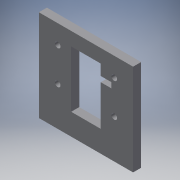
# Autodesk Inventor part: Camera holder plate
Saved by Autodesk Inventor 2018 (Build 220112000, 112)
## iProperties
Created: 2018-06-25
Part Number: Camera holder plate
Material: Generic
Document SubType Name: Modeling
Designer: Ajith Thomas
Density: 1 g/cm^3
Appearance: Default
Author: Ajith Thomas
Autodesk Inventor part; units mm, degrees
ref_plane "YZ Plane" through (0, 0, 0) normal (1, 0, 0) x (0, 1, 0)
ref_plane "XZ Plane" through (0, 0, 0) normal (0, 1, 0) x (-1, 0, 0)
ref_plane "XY Plane" through (0, 0, 0) normal (0, 0, 1) x (1, 0, 0)
sketch "Sketch1" plane through (0, 0, 0) normal (0, 0, 1) x (1, 0, 0)
  line L0 (-17.5, 19.5) -> (17.5, 19.5)
  line L1 (17.5, 19.5) -> (17.5, -14.5)
  line L2 (17.5, -14.5) -> (-17.5, -14.5)
  line L3 (-17.5, -14.5) -> (-17.5, 19.5)
  line L4 (-12.5, 14.5) -> (-12.5, -9.5) construction
  line L5 (12.5, 14.5) -> (-12.5, 14.5) construction
  line L6 (12.5, -9.5) -> (12.5, 14.5) construction
  line L7 (-12.5, -9.5) -> (12.5, -9.5) construction
  line L8 (8.7, 9.1) -> (8.7, 9.9) construction
  line L9 (8.7, 9.9) -> (7.48, 9.9) construction
  line L10 (7.48, 9.9) -> (7.48, 9.1) construction
  line L11 (7.48, 9.1) -> (8.7, 9.1) construction
  circle A0 centre (-10.5, 12.5) radius 1.05 projected
  circle A1 centre (-10.5, 0) radius 1.05 projected
  circle A2 centre (10.5, 12.5) radius 1.05 projected
  circle A3 centre (10.5, 0) radius 1.05 projected
  line L12 (-5.5, 14.5) -> (-5.5, -6.5)
  line L13 (-5.5, -6.5) -> (5.5, -6.5)
  line L14 (5.5, -6.5) -> (5.5, 8.5)
  line L15 (5.5, 8.5) -> (9.45, 8.5)
  line L16 (9.45, 8.5) -> (9.45, 10.5)
  line L17 (9.45, 10.5) -> (5.5, 10.5)
  line L18 (5.5, 10.5) -> (5.5, 14.5)
  line L19 (-5.5, 14.5) -> (5.5, 14.5)
  point P0 (0, 0)
  dimension "d0" = 5
  dimension "d1" = 5
  dimension "d2" = 35
  dimension "d3" = 5
  dimension "d4" = 5
  dimension "d5" = 7
  dimension "d6" = 7
  dimension "d7" = 3
  dimension "d8" = 18
  dimension "d9" = 3.05
  dimension "d10" = 4
  constraints: 24 end point, 6 perpendicular, 4 point on line, 2 parallel, 1 collinear, 1 horizontal, 1 vertical
  measures "d0" distance between parallel lines of L3 L4
  measures "d1" distance between parallel lines of L1 L6
  measures "d2" distance between parallel lines of L1 L3
  measures "d3" distance between parallel lines of L0 L5
  measures "d4" distance between parallel lines of L2 L7
  measures "d5" distance between parallel lines of L4 L12
  measures "d6" distance between parallel lines of L6 L14
  measures "d7" distance between parallel lines of L7 L13
  measures "d8" distance between parallel lines of L7 L15
  measures "d9" distance between parallel lines of L6 L16
  measures "d10" distance between parallel lines of L5 L17
extrude "Extrusion1" add sketch "Sketch1" along normal blind 3
sketch "Sketch2" plane through (0, 0, 3) normal (0, 0, 1) x (1, 0, 0)
  line L0 (-17.5, -14.5) -> (17.5, -14.5) construction
  line L1 (-17.5, 19.5) -> (-17.5, -14.5) construction
  line L2 (17.5, -14.5) -> (17.5, 19.5) construction
  line L3 (-17.5, -14.5) -> (17.5, -14.5)
  line L4 (17.5, -14.5) -> (17.5, -45.5)
  line L5 (17.5, -45.5) -> (-17.5, -45.5)
  line L6 (-17.5, -45.5) -> (-17.5, -14.5)
  line L7 (-12.5, -16.5) -> (-12.5, -40.5) construction
  line L8 (12.5, -40.5) -> (12.5, -16.5) construction
  line L9 (12.5, -16.5) -> (-12.5, -16.5) construction
  line L10 (-12.5, -40.5) -> (12.5, -40.5) construction
  line L11 (-7.3, -17.5) -> (7.3, -17.5)
  line L12 (7.3, -17.5) -> (7.3, -37.5)
  line L13 (7.3, -37.5) -> (-7.3, -37.5)
  line L14 (-7.3, -37.5) -> (-7.3, -17.5)
  circle A0 centre (-10.5, -26) radius 1.05 projected
  circle A1 centre (-10.5, -38.5) radius 1.05 projected
  circle A2 centre (10.5, -26) radius 1.05 projected
  circle A3 centre (10.5, -38.5) radius 1.05 projected
  point P0 (0, 0)
  dimension "d13" = 5
  dimension "d14" = 1
  dimension "d15" = 5.2
  dimension "d16" = 5.2
  dimension "d17" = 3
  constraints: 16 end point, 4 parallel, 2 horizontal, 2 perpendicular
  measures "d13" distance between parallel lines of L5 L10
  measures "d14" distance between parallel lines of L9 L11
  measures "d15" distance between parallel lines of L7 L14
  measures "d16" distance between parallel lines of L8 L12
  measures "d17" distance between parallel lines of L10 L13
extrude "Extrusion2" add sketch "Sketch2" against normal blind 3
sketch "Sketch3" plane through (0, 0, 3) normal (0, 0, 1) x (1, 0, 0)
  line L0 (17.5, 19.5) -> (17.5, -45.5) projected
  line L1 (-17.5, 19.5) -> (-17.5, -45.5) projected
  line L2 (-17.5, -45.5) -> (-17.5, 19.5) construction
  line L3 (-17.5, -13) -> (17.5, -13) construction
  line L4 (17.5, 19.5) -> (17.5, -45.5) construction
  line L5 (17.5, 1) -> (32.5, 1)
  line L6 (32.5, 1) -> (32.5, -27)
  line L7 (32.5, -27) -> (17.5, -27)
  line L8 (17.5, -27) -> (17.5, 1)
  line L9 (32.5, -8) -> (35.5, -8)
  line L10 (35.5, -8) -> (35.5, -18)
  line L11 (35.5, -18) -> (32.5, -18)
  line L12 (32.5, -18) -> (32.5, -8)
  line L13 (17.5, -13) -> (35.5, -13) construction
  point P0 (0, 0)
  dimension "d20" = 15
  dimension "d21" = 14
  dimension "d22" = 14
  dimension "d23" = 3
  dimension "d24" = 5
  dimension "d25" = 5
  constraints: 20 end point, 4 parallel, 3 midpoint, 3 perpendicular, 2 horizontal, 2 point on line
  measures "d20" distance of L6.end L7.end
  measures "d21" distance between parallel lines of L7 L3
  measures "d22" distance between parallel lines of L3 L5
  measures "d23" distance between parallel lines of L6 L10
  measures "d24" distance between parallel lines of L9 L13
  measures "d25" distance between parallel lines of L13 L11
extrude "Extrusion3" add sketch "Sketch3" against normal blind 3
ref_plane "Work Plane1" through (0, 19.5, 3) normal (1, 0, 0) x (0, 0, -1)
mirror "Mirror1" about plane through (0, 19.5, 3) normal (1, 0, 0) of "Extrusion3"
sketch "Sketch4" plane through (0, 0, 3) normal (0, 0, 1) x (1, 0, 0)
  circle A0 centre (22.6, -4) radius 1.8 projected
  circle A1 centre (22.6, -22) radius 1.8 projected
  circle A2 centre (-22.6, -22) radius 1.8 projected
  circle A3 centre (-22.6, -4) radius 1.8 projected
  point P0 (0, 0)
extrude "Extrusion4" cut sketch "Sketch4" against normal blind 14.1125
body "Solid1"
